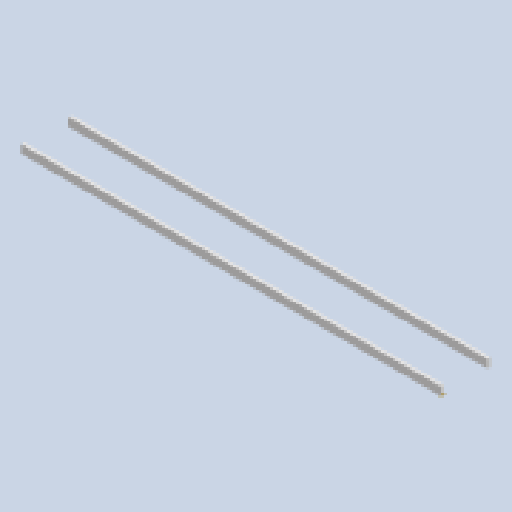
# Autodesk Inventor part: брусок
Saved by Autodesk Inventor 2024.2 (Build 282272000, 272)
## iProperties
Created: 2025-11-16
Part Number: брусок
Material: Типовые
Document SubType Name: Modeling
Designer: katya_notebook
Density: 1 g/cm^3
Appearance: По умолчанию
Author: katya_notebook
Autodesk Inventor part; units mm, degrees
ref_plane "YZ Plane" through (0, 0, 0) normal (1, 0, 0) x (0, 1, 0)
ref_plane "XZ Plane" through (0, 0, 0) normal (0, 1, 0) x (-1, 0, 0)
ref_plane "РабПлоскость2" through (1272.2614, -25.1804, 198.6497) normal (1, 0, 0) x (0, -1, 0)
sketch "Эскиз2" plane through (1272.2614, -25.1804, 198.6497) normal (1, 0, 0) x (0, -1, 0)
  line L0 (-3, -16) -> (0, -16) projected
  line L1 (0, 226) -> (0, -16) projected
  line L2 (0, -16) -> (-40, -16)
  line L3 (-40, -16) -> (-40, 0)
  line L4 (-40, 0) -> (0, 0)
  line L5 (0, 0) -> (0, -16)
  line L6 (0, 226) -> (-40, 226)
  line L7 (-40, 226) -> (-40, 210)
  line L8 (-40, 210) -> (0, 210)
  line L9 (0, 210) -> (0, 226)
  point P0 (-25.1804, 198.6497)
  point P1 (0, 0)
  dimension "d0" = 16
  dimension "d1" = 40
  dimension "d4" = 16
  dimension "d5" = 40
  constraints: 16 end point, 4 parallel, 2 horizontal, 2 perpendicular
  measures "d0" distance of L2.end L3.end
  measures "d1" distance of L0.end L2.end
  measures "d4" distance of L6.end L7.end
  measures "d5" distance of L7.end L8.end
ref_plane "РабПлоскость3" through (-738.3586, -22.1804, 198.6497) normal (-1, 0, 0) x (0, 0, 1)
extrude "Выдавливание1" add sketch "Эскиз2" against normal up to surface (2010.62 mm away)
